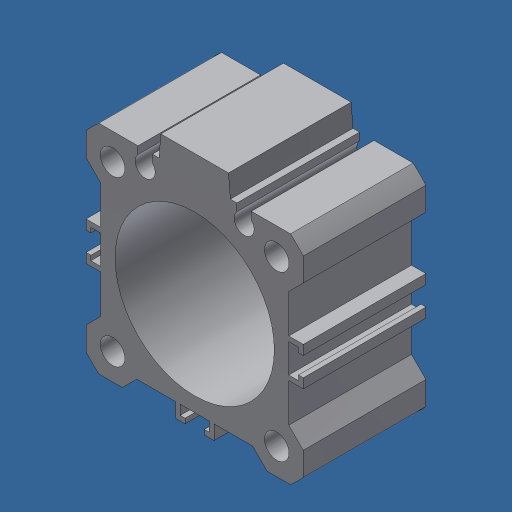
# Autodesk Inventor part: EXTRUSION, CYLINDER, ALUMINIUM, SMC, 32MM
Saved by Autodesk Inventor 2024.3 (Build 283343000, 343)
## iProperties
Category: _
Manager: _
Shininess: 64.0
Angle Display Precision: 2
Document Length Units: 11272
Document Angle Units: 11279
Document Time Units: 11290
Document Mass Units: 11286
Document Length Units Precision: 3
Document Angle Units Precision: 2
Part Number: EXTRUSION, CYLINDER, ALUMINIUM, SMC, 32MM
Material: Extrusion, Aluminum, SMC, 32 MM
Document SubType Name: Modeling
Created: 2019-07-31
Designer: -
Manufacturer: Standard
Standards Organization: Custom
Density: 2.71 g/cm^3
Mass: 61.0045 g
Surface Area: 125.663 cm^2
Volume: 22.5109 cm^3
Checked By: 00
Engr Approved By: _
User Status: Work In Process
Description: EXTRUSION, CYLINDER, ALUMINIUM, SMC, 32MM
Mfg Approved By: -
Appearance: Aluminum - Flat
ILogicPurgeVersion: 2.2.20.20
Density: 0.0
Volumn: 0.0
Area: 0.0
PropertySet Name: Model Information
Control State: 0
Master: False
Checked Out: False
CN_MASS: 0.06
CN_SERVICEABLE: _
CL_runCount: 0
FIRST_DESCRIPTION: _
SECOND_DESCRIPTION: _
THIRD_DESCRIPTION: _
ModelCat: Uncategorized
Author: -
Subject: _
Revision Number: A
Keywords: -
Autodesk Inventor part; units mm, degrees
ref_plane "YZ Plane" through (0, 0, 0) normal (1, 0, 0) x (0, 1, 0)
ref_plane "XZ Plane" through (0, 0, 0) normal (0, 1, 0) x (-1, 0, 0)
ref_plane "XY Plane" through (0, 0, 0) normal (0, 0, 1) x (1, 0, 0)
sketch "Sketch1" plane through (0, 0, 0) normal (0, 0, 1) x (1, 0, 0)
  circle A0 centre (0, 0) radius 16.5
  arc A1 (-19.8431, 22.5) -> (-22.5, 19.8431) centre (0, 0) ccw
  arc A2 (22.5, 19.8431) -> (19.8431, 22.5) centre (0, 0) ccw
  arc A3 (-22.5, -19.8431) -> (-19.8431, -22.5) centre (0, 0) ccw
  arc A4 (19.8431, -22.5) -> (22.5, -19.8431) centre (0, 0) ccw
  line L0 (-22.5, -15) -> (-19.5, -12)
  line L1 (-19.5, 12) -> (-22.5, 15)
  line L2 (-15, -22.5) -> (-12, -19.5)
  line L3 (12, -19.5) -> (15, -22.5)
  line L4 (22.5, -15) -> (19.5, -12)
  line L5 (19.5, 12) -> (22.5, 15)
  line L6 (-22.5, -19.8431) -> (-22.5, -15)
  line L7 (-22.5, 15) -> (-22.5, 19.8431)
  line L8 (19.8431, -22.5) -> (15, -22.5)
  line L9 (-15, -22.5) -> (-19.8431, -22.5)
  line L10 (22.5, 19.8431) -> (22.5, 15)
  line L11 (22.5, -15) -> (22.5, -19.8431)
  line L12 (19.5, 4) -> (22.5, 4)
  line L13 (22.5, 4) -> (22.5, 2)
  line L14 (22.5, 2) -> (21.5, 2)
  line L15 (21.5, 2) -> (21.5, 3)
  line L16 (21.5, 3) -> (19.5, 3)
  line L17 (19.5, -4) -> (22.5, -4)
  line L18 (22.5, -4) -> (22.5, -2)
  line L19 (22.5, -2) -> (21.5, -2)
  line L20 (21.5, -2) -> (21.5, -3)
  line L21 (21.5, -3) -> (19.5, -3)
  line L22 (4, -19.5) -> (4, -22.5)
  line L23 (4, -22.5) -> (2, -22.5)
  line L24 (2, -22.5) -> (2, -21.5)
  line L25 (2, -21.5) -> (3, -21.5)
  line L26 (3, -21.5) -> (3, -19.5)
  line L27 (-3, -19.5) -> (-3, -21.5)
  line L28 (-3, -21.5) -> (-2, -21.5)
  line L29 (-2, -21.5) -> (-2, -22.5)
  line L30 (-2, -22.5) -> (-4, -22.5)
  line L31 (-4, -22.5) -> (-4, -19.5)
  line L32 (-19.5, -4) -> (-22.5, -4)
  line L33 (-22.5, -4) -> (-22.5, -2)
  line L34 (-22.5, -2) -> (-21.5, -2)
  line L35 (-21.5, -2) -> (-21.5, -3)
  line L36 (-21.5, -3) -> (-19.5, -3)
  line L37 (-19.5, 4) -> (-22.5, 4)
  line L38 (-22.5, 4) -> (-22.5, 2)
  line L39 (-22.5, 2) -> (-21.5, 2)
  line L40 (-21.5, 2) -> (-21.5, 3)
  line L41 (-21.5, 3) -> (-19.5, 3)
  line L42 (-12, -19.5) -> (-4, -19.5)
  line L43 (-3, -19.5) -> (3, -19.5)
  line L44 (4, -19.5) -> (12, -19.5)
  line L45 (-19.5, -12) -> (-19.5, -4)
  line L46 (-19.5, -3) -> (-19.5, 3)
  line L47 (-19.5, 4) -> (-19.5, 12)
  line L48 (19.5, -12) -> (19.5, -4)
  line L49 (19.5, -3) -> (19.5, 3)
  line L50 (19.5, 4) -> (19.5, 12)
  line L51 (-7.3937, 22.5) -> (-7, 27)
  line L52 (-7, 27) -> (7, 27)
  line L53 (7, 27) -> (7.3937, 22.5)
  arc A5 (-11.75, 20.9337) -> (-8.75, 20.9337) centre (-10.25, 19.5) ccw
  arc A6 (8.75, 20.9337) -> (11.75, 20.9337) centre (10.25, 19.5) ccw
  line L54 (-8.75, 20.9337) -> (-8.75, 22.5)
  line L55 (-11.75, 20.9337) -> (-11.75, 22.5)
  line L56 (8.75, 20.9337) -> (8.75, 22.5)
  line L57 (-19.8431, 22.5) -> (-11.75, 22.5)
  line L58 (-8.75, 22.5) -> (-7.3937, 22.5)
  line L59 (11.75, 20.9337) -> (11.75, 22.5)
  line L60 (7.3937, 22.5) -> (8.75, 22.5)
  line L61 (11.75, 22.5) -> (19.8431, 22.5)
  point P0 (-17, 17)
  point P1 (17, 17)
  point P2 (17, -17)
  point P3 (-17, -17)
  dimension "d0" = 33
  dimension "d7" = 30
  dimension "d8" = 30
  dimension "d9" = 30
  dimension "d10" = 30
  dimension "d14" = 30
  dimension "d15" = 15
  dimension "d16" = 15
  dimension "d19" = 22.5
  dimension "d22" = 8
  dimension "d23" = 4
  dimension "d24" = 2
  dimension "d25" = 1
  dimension "d27" = 1
  dimension "d28" = 3
  dimension "d29" = 4
  dimension "d30" = 8
  dimension "d31" = 19.5
  dimension "d32" = 19.5
  dimension "d33" = 19.5
  dimension "d34" = 17
  dimension "d35" = 17
  dimension "d36" = 17
  dimension "d37" = 17
  dimension "d38" = 14
  dimension "d39" = 7
  dimension "d40" = 14.7874
  dimension "d42" = 7.3937
  dimension "d47" = 4.15
  dimension "d48" = 20.5
  dimension "d49" = 10.25
  dimension "d51" = 1.5
  dimension "d56" = 1.5
  dimension "d57" = 3
  dimension "d58" = 22.5
  dimension "d59" = 4.5
  constraints: 124 end point, 51 parallel, 49 perpendicular, 28 equal length, 14 horizontal alignment, 12 point on circle, 7 centre point, 7 vertical alignment, 4 horizontal, 2 coincident, 1 collinear, 1 equal radius
  measures "d0" diameter of A0
  measures "d7" radius of A1
  measures "d8" radius of A2
  measures "d9" radius of A4
  measures "d10" radius of A3
  measures "d14" distance of L0.start L1.end
  measures "d15" vertical distance of point (0, 0) L0.start
  measures "d16" horizontal distance of A0.centre L2.start
  measures "d19" distance from line of point (0, 0) L11
  measures "d22" distance between parallel lines of L17 L12
  measures "d23" distance from line of point (0, 0) L17
  measures "d24" distance of L12.end L13.end
  measures "d25" distance of L13.end L14.end
  measures "d27" distance between parallel lines of L12 L16
  measures "d28" distance of L17.start L17.end
  measures "d29" distance from line of point (0, 0) L22
  measures "d30" distance from line of L22.end L31
  measures "d31" distance from line of L48 point (0, 0)
  measures "d32" distance from line of point (0, 0) L47
  measures "d33" distance from line of point (0, 0) L42
  measures "d34" horizontal distance of point (0, 0) point (-17, 17)
  measures "d35" horizontal distance of point (0, 0) point (-17, -17)
  measures "d36" horizontal distance of point (17, 17) point (0, 0)
  measures "d37" horizontal distance of point (0, 0) point (17, 17)
  measures "d38" distance of L51.end L52.end
  measures "d39" horizontal distance of L52.end point (0, 0)
  measures "d40" distance of L53.end L51.start
  measures "d42" horizontal distance of point (0, 0) L51.start
  measures "d47" diameter of A5
  measures "d48" distance of A6.centre A5.centre
  measures "d49" horizontal distance of point (0, 0) A5.centre
  measures "d51" distance from line of A5.centre L54
  measures "d56" horizontal distance of A5.centre L55.start
  measures "d57" distance from line of A5.centre L57
  measures "d58" distance from line of L61 point (0, 0)
  measures "d59" distance between parallel lines of L52 L57
extrude "SMC, 32MM" add sketch "Sketch1" along normal blind 25.4
hole "Hole1" at (-17, 17, 0) at (17, 17, 0) at (17, -17, 0) at (-17, -17, 0) direction (0, 0, 1) diameter 5.1054 end through all
equation "\"d16\" = d15"
equation "\"d23\" = 0.5 * d22"
equation "\"d27\" = d25"
equation "\"d29\" = 0.5 * d22"
equation "\"d30\" = d22"
equation "\"d32\" = d31"
equation "\"d35\" = d34"
equation "\"d36\" = d34"
equation "\"d37\" = d35"
equation "\"d39\" = 0.5 * d38"
equation "\"d11\" = d5"
equation "\"d12\" = d6"
equation "\"d5\" = 22.5"
equation "\"d6\" = 22.5"
